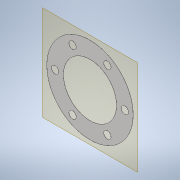
# Autodesk Inventor part: 垫片1
Saved by Autodesk Inventor 2020 (Build 240168000, 168)
## iProperties
Created: 2021-06-19
Part Number: 垫片1
Material: 常规
Document SubType Name: Modeling
Designer: dell
Density: 1 g/cm^3
Appearance: 默认
Author: dell
Autodesk Inventor part; units mm, degrees
ref_plane "YZ Plane" through (0, 0, 0) normal (1, 0, 0) x (0, 1, 0)
ref_plane "XZ Plane" through (0, 0, 0) normal (0, 1, 0) x (-1, 0, 0)
ref_plane "XY Plane" through (0, 0, 0) normal (0, 0, 1) x (1, 0, 0)
ref_plane "工作平面1" through (0, 0, 0) normal (0, 0, 1) x (1, 0, 0)
sketch "草图1" plane through (0, 0, 0) normal (0, 0, 1) x (1, 0, 0)
  circle A0 centre (0, 0) radius 40 projected
  circle A1 centre (0, 0) radius 65 projected
  circle A2 centre (-26.25, -45.4663) radius 5.5 projected
  circle A3 centre (-26.25, 45.4663) radius 5.5 projected
  circle A4 centre (26.25, -45.4663) radius 5.5 projected
  circle A5 centre (52.5, 0) radius 5.5 projected
  circle A6 centre (-52.5, 0) radius 5.5 projected
  circle A7 centre (26.25, 45.4663) radius 5.5 projected
  point P0 (0, 0)
extrude "拉伸1" add sketch "草图1" along normal blind 0.15
